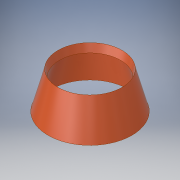
# Autodesk Inventor part: phenolic_bottom
Saved by Autodesk Inventor 2017 SP1 (Build 210196100, 196)
## iProperties
Created: 2016-07-25
Part Number: phenolic_bottom
Material: Phenolic Resin
Document SubType Name: Modeling
Designer: Jared
Density: 1.38 g/cm^3
Appearance: Smooth - Light Orange
Author: Jared
Autodesk Inventor part; units mm, degrees
ref_plane "YZ Plane" through (0, 0, 0) normal (1, 0, 0) x (0, 1, 0)
ref_plane "XZ Plane" through (0, 0, 0) normal (0, 1, 0) x (-1, 0, 0)
ref_plane "XY Plane" through (0, 0, 0) normal (0, 0, 1) x (1, 0, 0)
sketch "Sketch1" plane through (0, 0, 0) normal (0, 0, 1) x (1, 0, 0)
  line L0 (0, 25.4) -> (-28.702, 25.4) construction
  line L1 (0, 25.4) -> (-95.25, 25.4) construction
  line L2 (-95.25, 25.4) -> (-89.1588, 25.4) construction
  line L3 (-89.1588, 25.4) -> (-85.693, 23.7839) construction
  line L4 (-89.1588, 25.4) -> (-89.1588, 21.1626) construction
  line L5 (-89.1588, 0) -> (-95.25, 0)
  line L6 (-28.702, 59.6457) -> (-28.702, -91.9304) construction
  arc A0 (-28.9184, -8.4804) -> (-32.3684, -1.0818) centre (-35.052, -6.8369) ccw
  line L7 (-89.1588, 25.4) -> (-89.1588, 0)
  line L8 (-89.1588, 25.4) -> (-32.3684, -1.0818)
  line L9 (-28.9184, -8.4804) -> (-28.9392, -8.5583)
  line L10 (0, -319.0244) -> (0, 122.7573) projected
  line L11 (-73.152, 17.9359) -> (-28.702, 17.9359) construction
  line L12 (-89.1588, 0) -> (-92.3338, 0)
  line L13 (11.4547, -6.8369) -> (-136.2084, -6.8369) construction
  line L14 (-57.2892, -89.8271) -> (-74.8171, -155.2422)
  line L15 (-92.3338, -12.7) -> (-73.2838, -12.7)
  line L16 (-73.2838, -12.7) -> (-54.421, -103.6575)
  line L17 (-74.8171, -155.2422) -> (-68.2431, -155.2422)
  line L18 (-92.3338, -25.4) -> (-79.6338, -25.4)
  line L19 (-79.6338, -25.4) -> (-79.6338, -57.15)
  line L20 (-79.6338, -57.15) -> (-72.991, -88.4936)
  line L21 (-92.3338, 0) -> (-92.3338, -25.4)
  line L22 (-86.3902, -25.4) -> (-86.3902, -31.3436)
  line L23 (-86.3902, -31.3436) -> (-92.3338, -31.3436)
  line L24 (-92.3338, -31.3436) -> (-92.3338, -56.7436)
  line L25 (-92.3338, -56.7436) -> (-79.6338, -56.7436)
  line L26 (-73.152, 17.9359) -> (-32.3684, -1.0818)
  line L27 (-73.152, 17.9359) -> (-50.7653, -90.0141)
  line L28 (-50.7653, -90.0141) -> (-28.9184, -8.4804)
  line L29 (-52.4654, -96.3589) -> (-28.9184, -8.4804)
  line L30 (-86.36, -222.8555) -> (-28.9184, -8.4804)
  line L31 (-72.991, -88.4936) -> (-89.535, -222.8555)
  line L32 (-89.535, -222.8555) -> (-86.36, -222.8555)
  point P0 (0, 0)
  point P1 (-95.25, -255.9127)
  point P2 (-88.7095, 22.4389)
  dimension "d0" = 28.702
  dimension "d3" = 25
  dimension "d5" = 25.4
  dimension "d6" = 25.4
  dimension "d8" = 12.7
  dimension "d34" = 15
  dimension "d37" = 44.45
  dimension "d46" = 19.05
  dimension "d47" = 12.7
  dimension "d55" = 12.7
  dimension "d56" = 31.75
  dimension "d58" = 0.25
  dimension "d60" = 12.7
  dimension "d61" = 25.4
  dimension "d62" = 5.9436
  dimension "d63" = 5.9436
  dimension "d64" = 3.175
  dimension "d68" = 107.95
  dimension "d69" = 6.35
  dimension "d70" = 6.35
  dimension "d71" = 3.175
  dimension "d73" = 86.36
  dimension "d74" = 31.75
  dimension "d75" = 6.3448
  constraints: 64 end point, 15 point on line, 7 horizontal, 7 perpendicular, 6 tangent, 4 vertical, 3 collinear, 3 vertical alignment, 2 parallel, 2 point on circle, 1 centre point, 1 horizontal alignment, 1 midpoint
  measures "d0" distance of L0.start L0.end
  measures "d3" angle of L1 L3
  measures "d5" distance of point (0, 0) L0.start
  measures "d6" distance of L2.end L5.start
  measures "d8" diameter of A0
  measures "d34" angle of L6 L9
  measures "d37" distance of L11.start L11.end
  measures "d46" distance of L15.start L15.end
  measures "d47" distance between parallel lines of L12 L15
  measures "d55" distance between parallel lines of L15 L18
  measures "d56" distance of L18.end L19.end
  measures "d58" angle of L16 L20
  measures "d60" distance between parallel lines of L21 L19
  measures "d61" distance of L23.end L24.end
  measures "d62" distance of L22.start L22.end
  measures "d63" distance between parallel lines of L21 L22
  measures "d64" distance between parallel lines of L7 L21
  measures "d68" vertical distance of L11.start L27.end
  measures "d69" distance between parallel lines of L16 L27
  measures "d70" distance between parallel lines of L30 L14
  measures "d71" distance of L31.end L30.start
  measures "d73" distance from line of L10 L30.start
  measures "d74" distance from line of L25 L20.end
  measures "d75" distance from line of L31 L14.end
revolve "Revolution3" add sketch "Sketch1" angle 360 about axis through (0, -10, 0) along (0, 1, 0) contours L16 L30 L17 L14
body "Solid3"
